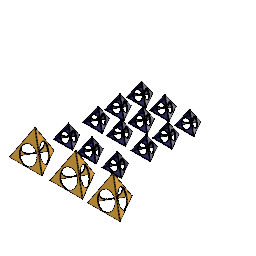
Painter Tripod Day#15 v3 (Autodesk Fusion 360 design; units mm, degrees)
Autodesk Fusion 360 part; units mm, degrees
sketch "Bottom Contour" plane through (0, 0, 0) normal (0, 0, 1) x (1, 0, 0) in component "60mm Painter's Tripod"
  line L0 (0, 0) -> (30, 51.9615)
  line L1 (30, 51.9615) -> (60, 0)
  line L2 (60, 0) -> (0, 0)
  dimension "d1" = 60
  constraint coincident L0.start L2.end
  constraint horizontal L2
  constraint equal L0 L1
  constraint equal L1 L2
  measures "d1" distance of L0.start L0.end
ref_plane "WorkPlane1" through (30, 25.9808, 50) normal (0, 0, 1) x (1, 0, 0) in component "60mm Painter's Tripod"
sketch "Top Point" plane through (30, 25.9808, 50) normal (0, 0, 1) x (1, 0, 0) in component "60mm Painter's Tripod"
  line L0 (-30, -25.9808) -> (0, 25.9808)
  line L1 (0, 25.9808) -> (30, -25.9808)
  line L2 (30, -25.9808) -> (-30, -25.9808)
  line L3 (0, 25.9808) -> (0, -25.9808) construction
  line L4 (-30, -25.9808) -> (15, 0) construction
  point P0 (0, -8.6603)
  constraint coincident L0.end L1.start
  constraint midpoint L2 L3.end
  constraint coincident L0.start L2.end
  constraint midpoint L1 L4.end
  constraint coincident L3 P0
  constraint coincident L4 P0
loft "Loft1" add profiles "Bottom Contour" section 1 section 2 point at (30, 17.3205, 50) makes body 1 in component "60mm Painter's Tripod"
shell "Shell1" thickness 2.5 removed faces 1 at (30, 17.3205, 0) on bodies 1 in component "60mm Painter's Tripod"
sketch "Sketch3" plane through (40.1786, 23.1971, 16.0714) normal (0.818317, 0.472456, 0.327327) x (-0.5, 0.866025, 0) in component "60mm Painter's Tripod"
  line L0 (-30, -17.0084) -> (30, -17.0084)
  line L1 (30, -17.0084) -> (0, 35.9066)
  line L2 (0, 35.9066) -> (-30, -17.0084)
  line L3 (0, 35.9066) -> (0, -17.0084) construction
  line L4 (-30, -17.0084) -> (15.4054, 8.734) construction
  circle A0 centre (0, 0) radius 12.5
  dimension "d4" = 25
  constraint coincident L1.end L2.start
  constraint midpoint L0 L3.end
  constraint coincident L0.start L2.end
  constraint coincident L1 L4.end
  constraint perpendicular L1 L4
  constraint coincident A0.centre origin
  measures "d4" diameter of A0
extrude "Extrude1" cut sketch "Sketch3" against normal up to surface (2.5 mm away) contours A0 bodies 1 in component "60mm Painter's Tripod"
pattern_circular "C-Pattern1" count 3 over 360 about axis through (30, 17.3205, 75) along (0, 0, -1) of "Extrude1" in component "60mm Painter's Tripod"
fillet "Fillet1" radius 1 3 edges at (45, 8.6603, 25) (30, 34.641, 25) (15, 8.6603, 25) on bodies 1 in component "60mm Painter's Tripod"
sketch "Bottom Contour (2)" plane through (0, 0, 0) normal (0, 0, 1) x (1, 0, 0) in component "100mm Painter's Tripod (1)"
  line L0 (0, 0) -> (50, 86.6025)
  line L1 (50, 86.6025) -> (100, 0)
  line L2 (100, 0) -> (0, 0)
  dimension "d1_1" = 100
  constraint coincident L0.start L2.end
  constraint horizontal L2
  constraint equal L0 L1
  constraint equal L1 L2
  measures "d1_1" distance of L0.start L0.end
ref_plane "WorkPlane1" through (50, 43.3013, 90) normal (0, 0, 1) x (1, 0, 0) in component "100mm Painter's Tripod (1)"
sketch "Top Point (2)" plane through (30, 25.9808, 90) normal (0, 0, 1) x (1, 0, 0) in component "100mm Painter's Tripod (1)"
  line L0 (-30, -25.9808) -> (20, 60.6218)
  line L1 (20, 60.6218) -> (70, -25.9808)
  line L2 (70, -25.9808) -> (-30, -25.9808)
  line L3 (20, 60.6218) -> (20, -25.9808) construction
  line L4 (-30, -25.9808) -> (45, 17.3205) construction
  point P0 (20, 2.8868)
  constraint coincident L0.end L1.start
  constraint midpoint L2 L3.end
  constraint coincident L0.start L2.end
  constraint midpoint L1 L4.end
  constraint coincident L3 P0
  constraint coincident L4 P0
loft "Loft1'" add profiles "Bottom Contour (2)" section 1 section 2 point at (50, 28.8675, 90) separate body makes body 2 in component "100mm Painter's Tripod (1)"
shell "Shell1'" thickness 2.5 removed faces 1 at (50, 28.8675, 0) on bodies 2 in component "100mm Painter's Tripod (1)"
sketch "Sketch3 (2)" plane through (68.0037, 39.262, 25.1866) normal (0.824644, 0.476108, 0.305424) x (-0.5, 0.866025, 0) in component "100mm Painter's Tripod (1)"
  line L0 (-50, -26.4505) -> (50, -26.4505)
  line L1 (50, -26.4505) -> (0, 68.0659)
  line L2 (0, 68.0659) -> (-50, -26.4505)
  line L3 (0, 68.0659) -> (0, -26.4505) construction
  line L4 (-50, -26.4505) -> (25, 20.8077) construction
  circle A0 centre (0, 0) radius 25
  dimension "d4_1" = 50
  constraint coincident L1.end L2.start
  constraint midpoint L0 L3.end
  constraint coincident L0.start L2.end
  constraint coincident L1 L4.end
  constraint coincident A0.centre origin
  constraint midpoint L1 L4.end
  measures "d4_1" diameter of A0
extrude "Extrude1'" cut sketch "Sketch3 (2)" against normal up to surface (2.5 mm away) contours A0 bodies 2 in component "100mm Painter's Tripod (1)"
pattern_circular "C-Pattern1'" count 3 over 360 about axis through (50, 28.8675, 125) along (0, 0, -1) of "Extrude1'" in component "100mm Painter's Tripod (1)"
fillet "Fillet1'" radius 1 3 edges at (75, 14.4338, 45) (50, 57.735, 45) (25, 14.4338, 45) on bodies 2 in component "100mm Painter's Tripod (1)"
move_body "Move1" bodies 2 to x (1, 0, 0) y (0, 1, 0) z (0, 0, 1) at (-5.889, -121.8234, -25.603) in component "100mm Painter's Tripod (1)"
pattern_linear "00000000-0000-0000-0000-000000000000" [suppressed]
pattern_linear "00000000-0000-0000-0000-000000000000'" [suppressed]
component "60mm Painter's Tripod" placed x (1, 0, 0) y (0, 1, 0) z (0, 0, 1) at (-65.9011, 27.8551, 0)
component "60mm Painter's Tripod" placed x (1, 0, 0) y (0, 1, 0) z (0, 0, 1) at (-65.124, 113.5212, 1.2359)
component "100mm Painter's Tripod (1)" placed x (1, 0, 0) y (0, 1, 0) z (0, 0, 1) at (6.9903, 38.7527, 23.3765)
component "100mm Painter's Tripod (1)" placed x (1, 0, 0) y (0, 1, 0) z (0, 0, 1) at (-105.0151, 38.6501, 25.3558)
component "60mm Painter's Tripod" placed x (1, 0, 0) y (0, 1, 0) z (0, 0, 1) at (-141.4519, 27.7303, -0.0955)
component "60mm Painter's Tripod" placed x (1, 0, 0) y (0, 1, 0) z (0, 0, 1) at (-141.3312, 115.7089, 0.9364)
component "100mm Painter's Tripod (1)" placed x (1, 0, 0) y (0, 1, 0) z (0, 0, 1) at (-225.4654, 37.7964, 25.8377)
component "60mm Painter's Tripod" placed x (1, 0, 0) y (0, 1, 0) z (0, 0, 1) at (-212.2632, 28.2523, -0.1909)
component "60mm Painter's Tripod" placed x (1, 0, 0) y (0, 1, 0) z (0, 0, 1) at (-211.1965, 116.0408, 0.1779)
component "60mm Painter's Tripod" placed x (1, 0, 0) y (0, 1, 0) z (0, 0, 1) at (-211.1965, 181.0408, 0.1779)
component "60mm Painter's Tripod" placed x (1, 0, 0) y (0, 1, 0) z (0, 0, 1) at (-141.3312, 180.7089, 0.9364)
component "60mm Painter's Tripod" placed x (1, 0, 0) y (0, 1, 0) z (0, 0, 1) at (-65.124, 178.5212, 1.2359)
component "60mm Painter's Tripod" placed x (1, 0, 0) y (0, 1, 0) z (0, 0, 1) at (-211.1965, 246.0408, 0.1779)
component "60mm Painter's Tripod" placed x (1, 0, 0) y (0, 1, 0) z (0, 0, 1) at (-141.3312, 245.7089, 0.9364)
component "60mm Painter's Tripod" placed x (1, 0, 0) y (0, 1, 0) z (0, 0, 1) at (-65.124, 243.5212, 1.2359)
